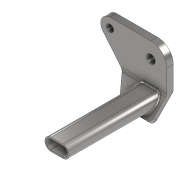
# Autodesk Inventor part: frame achterkant links
Saved by Autodesk Inventor 2020.3 (Build 243373000, 373)
## iProperties
Created: 2020-09-15
Part Number: frame achterkant links
Material: Stainless Steel
Document SubType Name: Modeling
Designer: Svend
Density: 8 g/cm^3
Appearance: Semi-Polished
Author: Svend
Autodesk Inventor part; units mm, degrees
ref_plane "YZ Plane" through (0, 0, 0) normal (1, 0, 0) x (0, 1, 0)
ref_plane "XZ Plane" through (0, 0, 0) normal (0, 1, 0) x (-1, 0, 0)
ref_plane "XY Plane" through (0, 0, 0) normal (0, 0, 1) x (1, 0, 0)
sketch "Sketch1" plane through (0, 0, 0) normal (0, 0, 1) x (1, 0, 0)
  line L0 (0, 8) -> (15.0435, 8)
  arc A0 (15.0435, -8) -> (15.0435, 8) centre (15.0435, 0) ccw
  arc A1 (0, 8) -> (0, -8) centre (0, 0) ccw
  line L1 (0, -8) -> (15.0435, -8)
  line L2 (15.0435, 6) -> (0, 6)
  arc A2 (0, 6) -> (0, -6) centre (0, 0) ccw
  line L3 (0, -6) -> (15.0435, -6)
  arc A3 (15.0435, -6) -> (15.0435, 6) centre (15.0435, 0) ccw
  dimension "d0" = 8
  dimension "d1" = 8
  dimension "d2" = 2
  constraints: 8 end point, 8 point on circle, 4 centre point, 3 tangent, 2 coincident, 1 horizontal, 1 horizontal alignment, 3 other
  measures "d0" radius of A1
  measures "d1" radius of A0
  measures "d2" distance between parallel lines of L0 L2
extrude "Extrusion1" add sketch "Sketch1" along normal blind 120
sketch "Sketch2" plane through (0, 0, 0) normal (1, 0, 0) x (0, 1, 0)
  line L0 (-8, 0) -> (-8, 120) projected
  line L1 (-6, 0) -> (6, 0) projected
  line L2 (8, 0) -> (8, 120) projected
  line L3 (8, 0) -> (-8, 0) projected
  line L4 (8, 0) -> (-8, 16)
  line L5 (-8, 16) -> (-8, 0)
  line L6 (8, 0) -> (-8, 0)
  point P0 (0, 0)
  dimension "d5" = 45
  constraints: 6 end point, 2 collinear, 1 point on line
  measures "d5" angle of L1 L4
extrude "Extrusion2" cut sketch "Sketch2" against normal through all both and the other way through all
sketch "Sketch3" plane through (15.0435, -8, 16) normal (0, -0.7071068, -0.7071068) x (-1, 0, 0)
  line L0 (15.0435, 19.799) -> (0, 19.799) projected
  ellipse E0 centre (15.0435, 11.3137) end of major axis (15.0435, 2.8284) minor radius 6 (15.0435, 2.8284) -> (15.0435, 19.799) ccw projected
  line L1 (0, 2.8284) -> (15.0435, 2.8284) projected
  ellipse E1 centre (0, 11.3137) end of major axis (0, 19.799) minor radius 6 (0, 19.799) -> (0, 2.8284) ccw projected
  ellipse E2 centre (0, 11.3137) end of major axis (0, 0) minor radius 8 (0, 22.6274) -> (0, 0) ccw projected
  line L2 (15.0435, 0) -> (0, 0) projected
  ellipse E3 centre (15.0435, 11.3137) end of major axis (15.0435, 22.6274) minor radius 8 (15.0435, 0) -> (15.0435, 22.6274) ccw projected
  line L3 (0, 22.6274) -> (15.0435, 22.6274) projected
  line L4 (0, 11.3137) -> (15.0435, 11.3137) construction
  line L5 (-12.4783, 28.8137) -> (27.5217, 28.8137)
  line L6 (27.5217, 28.8137) -> (27.5217, -6.1863)
  line L7 (27.5217, -6.1863) -> (-12.4783, -6.1863)
  line L8 (-12.4783, -6.1863) -> (-12.4783, 28.8137)
  line L9 (-12.4783, 28.8137) -> (27.5217, -6.1863) construction
  line L10 (27.5217, 28.8137) -> (-12.4783, -6.1863) construction
  line L11 (-12.4783, -6.1863) -> (-32.6855, 28.8137)
  line L12 (-32.6855, 28.8137) -> (-12.4783, 28.8137)
  point P0 (15.0435, 16.9706)
  point P1 (7.5217, 11.3137)
  dimension "d8" = 40
  dimension "d9" = 35
  dimension "d13" = 30
  constraints: 18 end point, 3 midpoint, 2 horizontal, 2 parallel, 1 collinear, 1 perpendicular, 4 other
  measures "d8" distance of L6.end L7.end
  measures "d9" distance of L5.end L6.end
  measures "d13" angle of L8 L11
extrude "Extrusion3" add sketch "Sketch3" along normal blind 6 contours E0 L1 E1 L0 | L3 E3 L2 E2 | L5 L6 L7 L8 | L8 L11 L12
sketch "Sketch4" plane through (-12.4783, -12.3744, 20.3744) normal (-1, 0, 0) x (0, 0.7071068, 0.7071068)
  line L0 (0, 0) -> (0, 35) projected
  line L1 (0, 35) -> (-6, 35) projected
  line L2 (-6, 0) -> (-6, 35) projected
  line L3 (0, 0) -> (-6, 0) projected
  line L4 (-6, 0) -> (-6, 35) projected
  line L5 (-6, 35) -> (0, 29)
  point P0 (-5.6569, 23.1569)
  dimension "d14" = 45
  constraints: 2 end point, 1 point on line
  measures "d14" angle of L1 L5
extrude "Extrusion4" cut sketch "Sketch4" against normal through all contours L5 L1 L0
sketch "Sketch5" plane through (-12.4783, 8.1317, -0.1317) normal (0, 1, 0) x (1, 0, 0)
  line L0 (60.2073, 8.4853) -> (56.7432, 0) projected
  line L1 (0, 8.4853) -> (60.2073, 8.4853) projected
  line L2 (0, 0) -> (0, 8.4853) projected
  line L3 (56.7432, 0) -> (0, 0) projected
  point P0 (12.4783, -0.1317)
extrude "Extrusion5" add sketch "Sketch5" along normal blind 50
fillet "Fillet1" radius 20 1 edges at (-12.4783, 58.1317, -4.3744)
sketch "Sketch6" plane through (-12.4783, 8.1317, -0.1317) normal (0, 0, 1) x (1, 0, 0)
  line L0 (56.7432, 0) -> (40, -20.5061) projected
  line L1 (56.7432, 0) -> (97.568, 50)
  line L2 (60.2073, 0) -> (40, -24.7487) projected
  line L3 (60.2073, 0) -> (60.2073, 50) projected
  line L4 (97.568, 50) -> (60.2073, 50)
  line L5 (20, 50) -> (56.7432, 50) projected
  line L6 (56.7432, 0) -> (50.1036, -8.1317)
  line L7 (60.2073, 50) -> (50.1036, 50)
  line L8 (50.1036, -8.1317) -> (50.1036, 50)
  point P0 (12.4783, -8.1317)
  constraints: 10 end point, 2 point on line, 1 collinear, 1 parallel, 1 perpendicular
extrude "Extrusion6" add sketch "Sketch6" against normal up to surface (8.4853 mm away)
sketch "Sketch7" plane through (-12.4783, -12.3744, 20.3744) normal (0, -0.7071068, 0.7071068) x (1, 0, 0)
  line L0 (50.1036, -6) -> (56.7432, -6) projected
  line L1 (50.1036, -6) -> (50.1036, -11.75) projected
  line L2 (50.1036, -11.75) -> (56.7432, -6) projected
  point P0 (12.4783, -5.6569)
extrude "Extrusion7" cut sketch "Sketch7" against normal through all
sketch "Sketch8" plane through (47.729, 8.1317, -8.617) normal (0, 0, -1) x (-1, 0, 0)
  line L0 (60.2073, 0) -> (0, 0) projected
  line L1 (60.2073, 0) -> (60.2073, 30) projected
  arc A0 (60.2073, 30) -> (40.2073, 50) centre (40.2073, 30) ccw projected
  line L2 (-37.3607, 50) -> (40.2073, 50) projected
  line L3 (0, 4.2426) -> (-37.3607, 50) projected
  line L4 (0, 0) -> (0, 4.2426) projected
  line L5 (0, 0) -> (0, 4.2426) projected
  line L6 (3.4641, 0) -> (20.2073, -20.5061) projected
  line L7 (0, 4.2426) -> (3.4641, 0)
  line L8 (3.4641, 0) -> (33.4863, -37.0053)
  line L9 (33.4863, -37.0053) -> (0, -37.0053)
  line L10 (0, -37.0053) -> (0, 4.2426)
  point P0 (47.729, -8.1317)
  constraints: 8 end point, 1 collinear, 1 perpendicular
extrude "Extrusion8" cut sketch "Sketch8" against normal through all contours L8 L9 L10 L0 | L0 L4 L7
fillet "Fillet2" radius 12 1 edges at (85.0897, 58.1317, -4.3744)
sketch "Sketch9" plane through (-12.4783, 8.1317, -0.1317) normal (0, 0, 1) x (1, 0, 0)
  arc A0 (81.5733, 30.4105) -> (72.2781, 50) centre (72.2781, 38) ccw projected
  line L0 (20, 50) -> (72.2781, 50) projected
  arc A1 (20, 50) -> (0, 30) centre (20, 30) ccw projected
  line L1 (0, 0) -> (0, 30) projected
  line L2 (56.7432, 0) -> (0, 0) projected
  line L3 (56.7432, 0) -> (81.5733, 30.4105) projected
  point P0 (12.4783, -8.1317)
hole "Hole1" at (7.5217, 38.1317, -0.1317) direction (0, 0, -1) diameter 11 depth 27.3 tip angle 118 clearance for "Countersunk Flat Head Screw ISO 2009/7046" size "M10" standard "ISO"
hole "Hole2" at (59.7998, 46.1317, -0.1317) direction (0, 0, -1) diameter 9 depth 27.3 tip angle 118 clearance for "Countersunk Flat Head Screw ISO 2009/7046" size "M8" standard "ISO"
fillet "Fillet3" radius 5 4 edges at (25.8541, -14.5614, 18.1873) (-12.4783, -14.4957, 18.253) (15.8933, 8.1317, -8.617) (15.8933, 8.1317, -0.1317)
fillet "Fillet4" radius 2 6 edges at (7.5217, -8, 16) (22.703, -2.3089, 10.3089) (17.3714, 7.6538, 0.5668) (7.5217, 8, 0.3797) (-2.3279, 7.6538, 0.5668) (-7.6596, -2.3089, 10.3089)
mirror "Mirror1" about plane through (0, 0, 0) normal (1, 0, 0) remove original yes
body "Solid1"
